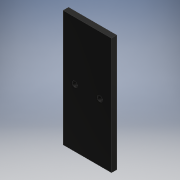
# Autodesk Inventor part: Hand Plate
Saved by Autodesk Inventor 2017 (Build 210142000, 142)
## iProperties
Created: 2018-10-18
Part Number: Hand Plate
Material: Generic
Document SubType Name: Modeling
Designer: Cameron
Density: 1 g/cm^3
Appearance: Glossy - Black
Author: Cameron
Autodesk Inventor part; units mm, degrees
ref_plane "YZ Plane" through (0, 0, 0) normal (1, 0, 0) x (0, 1, 0)
ref_plane "XZ Plane" through (0, 0, 0) normal (0, 1, 0) x (-1, 0, 0)
ref_plane "XY Plane" through (0, 0, 0) normal (0, 0, 1) x (1, 0, 0)
sketch "Sketch1" plane through (0, 0, 0) normal (0, 1, 0) x (-1, 0, 0)
  line L0 (0, 0) -> (27, 0)
  line L1 (27, 0) -> (27, -65)
  line L2 (27, -65) -> (0, -65)
  line L3 (0, -65) -> (0, 0)
  dimension "d0" = 27
  dimension "d1" = 65
  constraints: 8 end point, 2 parallel, 1 horizontal, 1 perpendicular
  measures "d0" distance of L1.end L2.end
  measures "d1" distance of L0.end L1.end
extrude "Extrusion1" add sketch "Sketch1" along normal blind 3
sketch "Sketch2" plane through (0, 3, 0) normal (0, 1, 0) x (1, 0, 0)
  line L0 (0, 0) -> (0, 65) projected
  line L1 (-27, 65) -> (-27, 0) projected
  line L2 (-27, 32.5) -> (0, 32.5)
  line L3 (-13.5, 32.5) -> (-20.5, 32.5)
  line L4 (-20.5, 32.5) -> (-6.5, 32.5)
  circle A0 centre (-20.5, 32.5) radius 1.5
  circle A1 centre (-6.5, 32.5) radius 1.5
  dimension "d4" = 7
  dimension "d5" = 14
  dimension "d6" = 3
  dimension "d7" = 3
  constraints: 6 end point, 3 midpoint, 2 centre point, 2 coincident, 2 point on line
  measures "d4" distance of L3.start L3.end
  measures "d5" distance of L3.end L4.end
  measures "d6" diameter of A0
  measures "d7" diameter of A1
extrude "Extrusion2" cut sketch "Sketch2" against normal blind 3
body "Solid1"
